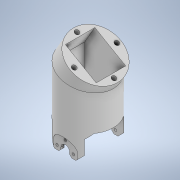
# Autodesk Inventor part: RL_spider_lower_leg_v3
Saved by Autodesk Inventor 2022 (Build 260153000, 153)
## iProperties
Created: 2021-08-10
Part Number: RL_spider_lower_leg_v3
Material: Generic
Document SubType Name: Modeling
Designer: Mock
Density: 1 g/cm^3
Appearance: Default
Author: Mock
Autodesk Inventor part; units mm, degrees
ref_plane "YZ Plane" through (0, 0, 0) normal (1, 0, 0) x (0, 1, 0)
ref_plane "XZ Plane" through (0, 0, 0) normal (0, 1, 0) x (-1, 0, 0)
sketch "Sketch2" plane through (0, 0, 0) normal (0, 0, 1) x (1, 0, 0)
  line L0 (0, 0) -> (0, 40)
  line L1 (0, 40) -> (7.5, 52.9904)
  dimension "d3" = 150
  dimension "d4" = 40
  dimension "d5" = 15
  constraints: 4 end point, 1 vertical
  measures "d3" angle of L0 L1
  measures "d4" distance of L0.start L0.end
  measures "d5" distance of L0.end L1.end
sketch "Sketch1" plane through (0, 0, 0) normal (0, 1, 0) x (-1, 0, 0)
  circle A0 centre (0, 0) radius 25
  line L0 (-17.5, -14.5) -> (17.5, -14.5)
  line L1 (17.5, -14.5) -> (17.5, 14.5)
  line L2 (17.5, 14.5) -> (-17.5, 14.5)
  line L3 (-17.5, 14.5) -> (-17.5, -14.5)
  arc A1 (17.5, -14.5) -> (17.5, 14.5) centre (0, 0) ccw
  arc A2 (-17.5, 14.5) -> (-17.5, -14.5) centre (0, 0) ccw
  dimension "d0" = 50
  dimension "d62" = 35
  dimension "d63" = 17.5
  dimension "d64" = 29
  dimension "d65" = 14.5
  constraints: 8 end point, 4 point on circle, 3 centre point, 2 parallel, 1 coincident, 1 horizontal, 1 perpendicular
  measures "d0" diameter of A0
  measures "d62" distance of L0.start L0.end
  measures "d63" distance from line of point (0, 0) L3
  measures "d64" distance of L2.end L0.start
  measures "d65" distance from line of point (0, 0) L0
sweep "Sweep1" add profiles "Sketch1" path "Sketch2" contours A0 | A2 L3 | L1 A1
sketch "Sketch3" plane through (0, 0, 0) normal (0, 0, 1) x (1, 0, 0)
  arc A0 (-7.2478, -27.2478) -> (7.2478, -27.2478) centre (0, -20) ccw
  line L0 (25, 0) -> (-25, 0) projected
  line L1 (25, 0) -> (-25, 0)
  line L2 (-25, 0) -> (-25, 46.6987) projected
  line L3 (-25, 0) -> (24.8538, 0)
  line L4 (24.8538, 0) -> (24.8538, -9.6419)
  line L5 (-25, -9.4957) -> (-25, 0)
  line L6 (24.8538, -9.6419) -> (7.2478, -27.2478)
  line L7 (-25, -9.4957) -> (-7.2478, -27.2478)
  point P0 (0, 0)
  point P1 (0, 0)
  dimension "d8" = 20.5
  dimension "d9" = 20
  dimension "d10" = 0
  dimension "d119" = 135
  dimension "d120" = 135
  constraints: 12 end point, 2 perpendicular, 2 point on circle, 2 tangent, 1 centre point, 1 coincident, 1 horizontal, 1 parallel
  measures "d8" diameter of A0
  measures "d9" distance from line of L0 A0.centre
  measures "d10" horizontal distance of A0.centre point (0, 0)
  measures "d119" angle of L7 L5
  measures "d120" angle of L4 L6
extrude "Extrusion2" add sketch "Sketch3" along normal mid plane 50
sketch "Sketch4" plane through (0, 0, 0) normal (0, 1, 0) x (-1, 0, 0)
  circle A0 centre (0, 0) radius 25
  circle A1 centre (0, 0) radius 40
  dimension "d112" = 50
  dimension "d113" = 80
  constraints: 2 centre point, 1 coincident
  measures "d112" diameter of A0
  measures "d113" diameter of A1
extrude "Extrusion3" cut sketch "Sketch4" against normal blind 50
sketch "Sketch5" plane through (0, 0, 0) normal (0, 0, 1) x (1, 0, 0)
  spline S0 degree 6 poles (-7.2478, -27.2478) (-6.8228, -27.6729) (-6.358, -28.0779) (-5.8519, -28.4591) (-5.3036, -28.8114) (-4.7124, -29.1287) (-3.8562, -29.5) (-3.629, -29.5911) (-3.3968, -29.6765) (-3.1599, -29.7559) (-2.9186, -29.829) (-2.5339, -29.9329) (-2.3936, -29.9683) (-2.252, -30.0015) (-2.1092, -30.0324) (-1.9653, -30.0609) (-1.5243, -30.1405) (-1.2238, -30.1839) (-0.9201, -30.2169) (-0.6142, -30.239) (-0.3072, -30.25) (0, -30.25) knots 0 0 0 0 0 0 0 0.511906 0.511906 0.511906 0.511906 0.511906 0.691167 0.691167 0.691167 0.691167 0.691167 0.792636 0.792636 0.792636 0.792636 0.792636 1 1 1 1 1 1 1 projected
  spline S1 degree 6 poles (0, -30.25) (0.0017, -30.25) (0.0033, -30.25) (0.005, -30.25) (0.0066, -30.25) (0.0083, -30.25) (0.318, -30.2497) (0.626, -30.2383) (0.9328, -30.2158) (1.2373, -30.1824) (1.5385, -30.1384) (1.9795, -30.0581) (2.1227, -30.0295) (2.2648, -29.9985) (2.4058, -29.9653) (2.5454, -29.9299) (2.9272, -29.8264) (3.1663, -29.7538) (3.4011, -29.6749) (3.6312, -29.5902) (3.8565, -29.4999) (4.7111, -29.1294) (5.3027, -28.8119) (5.8513, -28.4595) (6.3576, -28.0783) (6.8227, -27.673) (7.2478, -27.2478) knots 0 0 0 0 0 0 0 0.001119 0.001119 0.001119 0.001119 0.001119 0.209106 0.209106 0.209106 0.209106 0.209106 0.310152 0.310152 0.310152 0.310152 0.310152 0.48788 0.48788 0.48788 0.48788 0.48788 1 1 1 1 1 1 1 projected
  line L0 (-25, -9.4957) -> (-25, 46.6987) projected
  line L1 (7.2478, -27.2478) -> (24.8538, -9.6419) projected
  line L2 (-25, 0) -> (24.8538, 0)
  line L3 (24.8538, 0) -> (24.8538, -9.6419)
  line L4 (-25, -10) -> (-25, 0)
  line L5 (-25, -9.4957) -> (-7.2478, -27.2478) projected
  constraints: 6 end point, 1 horizontal, 1 parallel, 1 perpendicular, 1 point on line, 7 other
extrude "Extrusion4" cut sketch "Sketch5" along normal mid plane 38.4
sketch "Sketch7" plane through (0, 0, 0) normal (0, 0, 1) x (1, 0, 0)
  arc A0 (-7.2478, -27.2478) -> (7.2478, -27.2478) centre (0, -20) ccw projected
  circle A1 centre (0, -20) radius 4.25
  circle A2 centre (-8, -20) radius 1.25
  line L0 (0, -20) -> (-8, -20)
  line L1 (0, -20) -> (-2.2147, -20)
  circle A3 centre (0, -28) radius 1.25
  circle A4 centre (8, -20) radius 1.25
  circle A5 centre (0, -12) radius 1.25
  point P0 (0, 0)
  point P1 (8.6286, -25.5326)
  point P2 (-8.6286, -25.5326)
  dimension "d26" = 8.5
  dimension "d41" = 2.5
  dimension "d57" = 0
  dimension "d60" = 360
  constraints: 5 centre point, 4 end point, 1 coincident, 1 horizontal, 9 other
  measures "d26" diameter of A1
  measures "d41" diameter of A2
  measures "d57" distance between parallel lines of L0 L1
extrude "Extrusion6" cut sketch "Sketch7" along normal mid plane 50
ref_plane "Work Plane1" through (0, 0, 25) normal (0, 0, 1) x (1, 0, 0)
sketch "Sketch8" plane through (0, 0, 25) normal (0, 0, 1) x (1, 0, 0)
  circle A0 centre (0, -20) radius 4.25 projected
  circle A1 centre (0, -20) radius 12.5
  point P0 (0, 0)
  dimension "d35" = 25
  constraints: 1 centre point, 1 coincident
  measures "d35" diameter of A1
extrude "Extrusion7" cut sketch "Sketch8" against normal blind 2.8
mirror "Mirror1" about plane through (0, 0, 0) normal (0, 0, 1) of "Extrusion7"
sketch "Sketch9" plane through (7.5, 52.9904, 0) normal (0.5, 0.8660254, 0) x (0, 0, -1)
  circle A0 centre (21, 0) radius 2.2
  circle A1 centre (0, 21) radius 2.2
  circle A2 centre (-21, 0) radius 2.2
  circle A3 centre (0, -21) radius 2.2
  point P0 (0, -20)
  point P1 (0, 0)
  dimension "d49" = 21
  dimension "d50" = 4.4
  dimension "d53" = 360
  constraints: 4 centre point, 9 other
  measures "d49" distance of A0.centre point (0, 0)
  measures "d50" diameter of A0
extrude "Extrusion8" cut sketch "Sketch9" against normal blind 7
chamfer "Chamfer4" distance 4.7 angle 45 2 edges at (0, 0, 19.2) (0, 0, -19.2)
sketch "Sketch14" plane through (0, -20, -22.2) normal (0, 0, -1) x (-1, 0, 0)
  line L0 (11.4961, -2.9996) -> (7.2478, -7.2478) projected
  line L1 (11.4961, -2.9996) -> (16.0112, 1.5156) projected
  line L2 (-7.2478, -7.2478) -> (-11.4961, -2.9996) projected
  line L3 (-16.0112, 1.5156) -> (-11.4961, -2.9996) projected
  arc A0 (-7.2478, -7.2478) -> (7.2478, -7.2478) centre (0, 0) ccw projected
  circle A1 centre (0, 0) radius 4.25 projected
  circle A2 centre (0, 0) radius 4.25 projected
  line L4 (4.25, 0) -> (4.25, -2)
  line L5 (4.25, -2) -> (6.3869, -4.1369)
  line L6 (6.3869, -4.1369) -> (10.3588, -4.1369)
  line L7 (7.2478, -7.2478) -> (11.4961, -2.9996) projected
  line L8 (0, 0) -> (0, -1.4392)
  line L9 (-4.25, 0) -> (-4.25, -2)
  line L10 (-4.25, -2) -> (-6.3869, -4.1369)
  line L11 (-6.3869, -4.1369) -> (-10.3588, -4.1369)
  point P0 (0, 20)
  point P1 (-10.3588, -4.1369)
  dimension "d114" = 2
  dimension "d115" = 135
  dimension "d116" = 135
  constraints: 14 end point, 4 symmetric about line, 3 vertical, 1 horizontal alignment, 1 perpendicular, 1 point on line, 1 other
  measures "d114" distance of L4.start L4.end
  measures "d115" angle of L6 L0
  measures "d116" angle of L5 L6
extrude "Extrusion12" cut sketch "Sketch14" against normal blind 50 contours L0 A0 L2 L11 L10 L9 A1 L4 L5 L6
equation "\"d116\" = d115"
equation "\"d63\" = 0.5 * d62"
equation "\"d65\" = 0.5 * d64"
body "Solid2"
